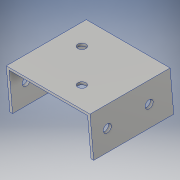
# Autodesk Inventor part: CAR_039_SweeperBarMount
Saved by Autodesk Inventor 2018.3 (Build 223284000, 284)
## iProperties
Created: 2020-02-16
Part Number: CAR_039_SweeperBarMount
Material: Aluminum 6061
Document SubType Name: Modeling
Designer: jd2
Density: 2.7 g/cm^3
Appearance: Aluminum - Flat
Author: jd2
Autodesk Inventor part; units mm, degrees
ref_plane "YZ Plane" through (0, 0, 0) normal (1, 0, 0) x (0, 1, 0)
ref_plane "XZ Plane" through (0, 0, 0) normal (0, 1, 0) x (-1, 0, 0)
ref_plane "XY Plane" through (0, 0, 0) normal (0, 0, 1) x (1, 0, 0)
sketch "Sketch5" plane through (0, 0, 0) normal (0, 0, 1) x (1, 0, 0)
  line L0 (1.6002, 0) -> (49.2125, 0)
  line L1 (50.8, 0) -> (50.8, 1.5875)
  line L2 (50.8, 1.5875) -> (0, 1.5875)
  line L3 (0, 1.5875) -> (0, 0)
  line L4 (50.8, 1.5875) -> (49.2125, 1.5875)
  line L5 (49.2125, 0) -> (49.2125, -23.8125)
  line L6 (49.2125, -23.8125) -> (50.8, -23.8125)
  line L7 (50.8, -23.8125) -> (50.8, 1.5875)
  line L8 (49.2125, 0) -> (49.2125, 1.5875)
  line L9 (0, 1.5875) -> (1.6002, 1.5875)
  line L10 (1.6002, 0) -> (1.6002, -23.8125)
  line L11 (1.6002, -23.8125) -> (0, -23.8125)
  line L12 (0, -23.8125) -> (0, 1.5875)
  dimension "d12" = 50.8
  dimension "d13" = 1.5875
  dimension "d14" = 25.4
  dimension "d15" = 1.5875
  dimension "d46" = 1.6002
  constraints: 26 end point, 6 parallel, 3 horizontal, 3 perpendicular, 1 vertical
  measures "d12" distance of L2.end L1.end
  measures "d13" distance of L1.start L1.end
  measures "d14" distance of L4.end L5.end
  measures "d15" distance between parallel lines of L7 L5
  measures "d46" distance of L10.end L11.end
extrude "Extrusion4" add sketch "Sketch5" along normal blind 50.8
sketch "Sketch6" plane through (50.8, -23.8125, 0) normal (1, 0, 0) x (0, 0, -1)
  line L0 (-50.8, 0) -> (-50.8, 25.4) projected
  line L1 (-50.8, 25.4) -> (-50.8, 0)
  line L2 (-50.8, 25.4) -> (-48.5778, 0)
  line L3 (-50.8, 23.8125) -> (-50.8, 0) projected
  line L4 (-48.5778, 0) -> (-50.8, 0)
  line L5 (0, 25.4) -> (-50.8, 25.4) projected
  point P0 (0, 23.8125)
  dimension "d18" = 85
  constraints: 6 end point, 1 collinear, 1 perpendicular
  measures "d18" angle of L5 L2
extrude "Extrusion5" cut sketch "Sketch6" against normal blind 228.6
sketch "Sketch7" plane through (50.8, -23.8125, 0) normal (1, 0, 0) x (0, 0, -1)
  line L0 (0, 0) -> (0, 25.4) projected
  line L1 (0, 25.4) -> (-50.8, 25.4) projected
  point P0 (0, 23.8125)
  point P1 (-40.3225, 12.7)
  point P2 (-14.9225, 12.7)
  dimension "d21" = 40.3225
  dimension "d22" = 14.9225
  dimension "d30" = 12.7
  dimension "d31" = 12.7
  measures "d21" distance from line of L0 point (-40.323, 12.7)
  measures "d22" distance from line of L0 point (-14.923, 12.7)
  measures "d30" distance from line of L1 point (-40.323, 12.7)
  measures "d31" distance from line of L1 point (-14.923, 12.7)
hole "Hole1" at (50.8, -11.1125, 40.3225) at (50.8, -11.1125, 14.9225) direction (-1, 0, 0) diameter 4.8514 end through all
sketch "Sketch8" plane through (50.8, -23.8125, 0) normal (1, 0, 0) x (0, 0, -1)
  line L0 (0, 0) -> (0, 25.4) projected
  line L1 (0, 0) -> (0, 25.4)
  line L2 (0, 25.4) -> (0, 0)
  line L3 (-2.2222, 25.4) -> (0, 0)
  line L4 (0, 25.4) -> (-50.8, 25.4) projected
  line L5 (-2.2222, 25.4) -> (0, 25.4)
  point P0 (0, 23.8125)
  dimension "d32" = 5
  constraints: 8 end point, 2 collinear, 1 vertical
  measures "d32" angle of L0 L3
extrude "Extrusion6" cut sketch "Sketch8" against normal blind 228.6
sketch "Sketch9" plane through (0, 1.5875, 50.6611) normal (0, -1, 0) x (1, 0, 0)
  line L0 (49.2125, 0) -> (1.6002, 0) projected
  line L1 (0, -50.6611) -> (0, -2.0833) projected
  point P0 (12.7, -33.02)
  point P1 (33.02, -12.7)
  dimension "d35" = 12.7
  dimension "d37" = 33.02
  dimension "d47" = 33.02
  dimension "d48" = 12.7
  measures "d35" distance from line of L0 point (33.02, -12.7)
  measures "d37" distance from line of L0 point (12.7, -33.02)
  measures "d47" distance from line of point (33.02, -12.7) L1
  measures "d48" distance from line of point (12.7, -33.02) L1
hole "Hole2" at (12.7, 1.5875, 17.6411) at (33.02, 1.5875, 37.9611) direction (0, -1, 0) diameter 4.8514 end through all
body "Solid2"
